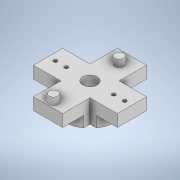
# Autodesk Inventor part: Adaptation_on_OPdevside_5_1
Saved by Autodesk Inventor 2022 (Build 260153000, 153)
## iProperties
Created: 2022-05-23
Part Number: Adaptation_on_OPdevside_5_1
Material: Generisch
Document SubType Name: Modeling
Designer: 123St
Density: 1 g/cm^3
Appearance: Vorgabe
Author: 123St
Autodesk Inventor part; units mm, degrees
ref_plane "YZ Plane" through (0, 0, 0) normal (1, 0, 0) x (0, 1, 0)
ref_plane "XZ Plane" through (0, 0, 0) normal (0, 1, 0) x (-1, 0, 0)
ref_plane "XY Plane" through (0, 0, 0) normal (0, 0, 1) x (1, 0, 0)
sketch "Skizze1" plane through (0, 0, 0) normal (0, 1, 0) x (-1, 0, 0)
  line L0 (11.5, 4) -> (4, 4)
  line L1 (-11.5, 4) -> (-11.5, -4)
  line L2 (-11.5, -4) -> (-4, -4)
  line L3 (11.5, -4) -> (11.5, 4)
  line L4 (4, 11.5) -> (-4, 11.5)
  line L5 (-4, 11.5) -> (-4, 4)
  line L6 (-4, -11.5) -> (4, -11.5)
  line L7 (4, -11.5) -> (4, -4)
  line L8 (4, 4) -> (4, 11.5)
  line L9 (4, -4) -> (11.5, -4)
  line L10 (-4, -4) -> (-4, -11.5)
  line L11 (-4, 4) -> (-11.5, 4)
  circle A0 centre (0, 0) radius 1.9807
  dimension "d0" = 8
  dimension "d1" = 8
  dimension "d2" = 8
  dimension "d3" = 8
  dimension "d4" = 4
  dimension "d5" = 4
  dimension "d6" = 23
  dimension "d7" = 23
  dimension "d8" = 11.5
  dimension "d9" = 11.5
  dimension "d10" = 4
  dimension "d11" = 4
  constraints: 24 end point, 10 parallel, 4 perpendicular, 3 horizontal, 1 centre point, 1 coincident
  measures "d0" distance of L3.start L0.start
  measures "d1" distance of L6.start L6.end
  measures "d2" distance of L1.start L1.end
  measures "d3" distance of L4.start L4.end
  measures "d4" distance from line of point (0, 0) L9
  measures "d5" distance from line of L7 point (0, 0)
  measures "d6" distance between parallel lines of L1 L3
  measures "d7" distance between parallel lines of L6 L4
  measures "d8" distance from line of point (0, 0) L4
  measures "d9" distance from line of L3 A0.centre
  measures "d10" distance from line of point (0, 0) L2
  measures "d11" distance from line of point (0, 0) L5
extrude "Extrusion1" add sketch "Skizze1" along normal blind 6.3
sketch "Skizze2" plane through (0, 6.3, 0) normal (0, 1, 0) x (1, 0, 0)
  circle A0 centre (0, -10) radius 1.2
  circle A1 centre (0, 8) radius 1.2
  point P0 (0, 0)
  dimension "d14" = 2.4
  dimension "d15" = 2.4
  dimension "d16" = 8
  dimension "d17" = 10
  constraints: 2 centre point
  measures "d14" diameter of A1
  measures "d15" diameter of A0
  measures "d16" distance of A1.centre point (0, 0)
  measures "d17" distance of point (0, 0) A0.centre
extrude "Extrusion2" add sketch "Skizze2" along normal blind 2
sketch "Skizze3" plane through (0, 6.3, 0) normal (0, 1, 0) x (1, 0, 0)
  circle A0 centre (-6.5, 0) radius 0.5
  circle A1 centre (-9.5, 0) radius 0.5
  circle A2 centre (6.5, 0) radius 0.5
  circle A3 centre (9.5, 0) radius 0.5
  point P0 (0, 0)
  dimension "d20" = 1
  dimension "d21" = 1
  dimension "d22" = 1
  dimension "d23" = 1
  dimension "d24" = 13
  dimension "d25" = 6.5
  dimension "d26" = 19
  dimension "d27" = 9.5
  constraints: 4 centre point
  measures "d20" diameter of A1
  measures "d21" diameter of A0
  measures "d22" diameter of A2
  measures "d23" diameter of A3
  measures "d24" distance of A2.centre A0.centre
  measures "d25" distance of point (0, 0) A0.centre
  measures "d26" distance of A3.centre A1.centre
  measures "d27" distance of point (0, 0) A1.centre
extrude "Extrusion3" cut sketch "Skizze3" against normal blind 10
sketch "Skizze4" plane through (0, 0, 0) normal (0, -1, 0) x (1, 0, 0)
  circle A0 centre (0, 0) radius 7
  circle A1 centre (0, 0) radius 22.2636
  dimension "d30" = 14
  constraints: 2 centre point, 2 coincident
  measures "d30" diameter of A0
extrude "Extrusion4" cut sketch "Skizze4" against normal blind 3
equation "\"d4\" = 0.5 * d0"
equation "\"d5\" = 0.5 * d1"
equation "\"d8\" = 0.5 * d7"
equation "\"d9\" = 0.5 * d6"
equation "\"d10\" = 0.5 * d2"
equation "\"d11\" = 0.5 * d3"
equation "\"d25\" = 0.5 * d24"
equation "\"d27\" = 0.5 * d26"
